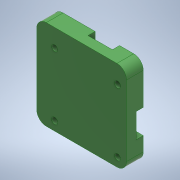
# Autodesk Inventor part: 071_0100_Base
Saved by Autodesk Inventor 2020 (Build 240168000, 168)
## iProperties
Created: 2018-07-06
Part Number: 071_0100_Base
Material: Generic
Document SubType Name: Modeling
Designer: deniz
Density: 1 g/cm^3
Appearance: Default
Author: deniz
Autodesk Inventor part; units mm, degrees
ref_plane "YZ Plane" through (0, 0, 0) normal (1, 0, 0) x (0, 1, 0)
ref_plane "XZ Plane" through (0, 0, 0) normal (0, 1, 0) x (-1, 0, 0)
ref_plane "XY Plane" through (0, 0, 0) normal (0, 0, 1) x (1, 0, 0)
sketch "Sketch1" plane through (0, 0, 0) normal (0, 1, 0) x (-1, 0, 0)
  line L0 (0, 0) -> (30, 0)
  line L1 (30, 0) -> (30, -30)
  line L2 (30, -30) -> (0, -30)
  line L3 (0, -30) -> (0, 0)
  line L4 (30, 0) -> (0, -30) construction
  line L5 (0, 0) -> (30, -30) construction
  line L6 (25.2, 0) -> (25.2, -4.8)
  line L7 (25.2, -4.8) -> (30, -4.8)
  line L8 (25.2, -25.2) -> (25.2, -30)
  line L9 (25.2, -25.2) -> (30, -25.2)
  line L10 (4.8, -25.2) -> (0, -25.2)
  line L11 (4.8, -25.2) -> (4.8, -30)
  line L12 (4.8, -4.8) -> (4.8, 0)
  line L13 (4.8, -4.8) -> (0, -4.8)
  line L14 (60, 30) -> (-15, 30)
  line L15 (-15, 30) -> (-15, -45)
  line L16 (-15, -45) -> (60, -45)
  line L17 (60, -45) -> (60, 30)
  circle A0 centre (45, 15) radius 5
  line L18 (25.2, 0) -> (25.2, 30)
  line L19 (30, -4.8) -> (60, -4.8)
  line L20 (4.8, 0) -> (4.8, 30)
  line L21 (0, -4.8) -> (-15, -4.8)
  line L22 (0, -25.2) -> (-15, -25.2)
  line L23 (4.8, -30) -> (4.8, -45)
  line L24 (25.2, -30) -> (25.2, -45)
  line L25 (30, -25.2) -> (60, -25.2)
  point P0 (-7.5, -37.5)
  point P1 (45, -37.5)
  point P2 (-7.5, 15)
  dimension "d0" = 30
  dimension "d1" = 30
  dimension "d2" = 20.4
  dimension "d7" = 30
  dimension "d8" = 30
  dimension "d9" = 15
  dimension "d10" = 15
  dimension "d11" = 15
  dimension "d12" = 15
  dimension "d13" = 10
  dimension "d14" = 7.5
  dimension "d15" = 7.5
  dimension "d18" = 15
  dimension "d19" = 7.5
  dimension "d20" = 7.5
  dimension "d21" = 15
  constraints: 52 end point, 31 point on line, 9 perpendicular, 4 parallel, 2 horizontal, 1 centre point, 1 coincident, 1 vertical
  measures "d0" distance of L1.end L2.end
  measures "d1" distance of L0.end L1.end
  measures "d2" distance between parallel lines of L9 L7
  measures "d7" distance between parallel lines of L1 L17
  measures "d8" distance between parallel lines of L14 L0
  measures "d9" distance between parallel lines of L16 L2
  measures "d10" distance between parallel lines of L15 L3
  measures "d11" distance from line of L17 A0.centre
  measures "d12" distance from line of L14 A0.centre
  measures "d13" diameter of A0
  measures "d14" distance from line of L16 point (-7.5, -37.5)
  measures "d15" distance from line of L15 point (-7.5, -37.5)
  measures "d18" distance from line of L14 point (-7.5, 15)
  measures "d19" distance from line of L15 point (-7.5, 15)
  measures "d20" distance from line of L16 point (45, -37.5)
  measures "d21" distance from line of L17 point (45, -37.5)
extrude "Extrusion1" add sketch "Sketch1" along normal blind 2 contours L20 L14 L18 L0 | L0 L6 L7 L1 L9 L8 L2 L11 L10 L3 L13 L12 | L3 L22 L15 L21 | L19 L17 L25 L1 | L2 L24 L16 L23
extrude "Extrusion2" add sketch "Sketch1" along normal blind 8 contours L3 L21 L15 L14 L20 L0 | L0 L12 L13 L3 | L18 L14 L17 L19 L1 L0 | L0 L1 L7 L6 | L10 L11 L2 L3 | L3 L2 L23 L16 L15 L22 | L25 L17 L16 L24 L2 L1 | L1 L2 L8 L9 | A0
hole "Hole1" at (-45, 0, -37.5) at (7.5, 0, 15) direction (0, 1, 0) diameter 5.2 depth 10 tip angle 118
hole "Hole2" at (-45, 0, 15) at (7.5, 0, -37.5) direction (0, 1, 0) diameter 4.95 depth 10 tip angle 118
fillet "Fillet1" radius 8 4 edges at (-60, 4, 30) (15, 4, 30) (15, 4, -45) (-60, 4, -45)
fillet "Fillet2" radius 2 1 edges at (-25.2, 5, -4.8)
move faces "Move1" translate (0, -6, 0) faces at (-10.5471, 0, -19.3825)
equation "\"d14\" = 0.5 * d9"
equation "\"d15\" = 0.5 * d10"
equation "\"d18\" = d12"
equation "\"d19\" = d15"
equation "\"d20\" = d14"
equation "\"d21\" = d11"
body "Solid1"
